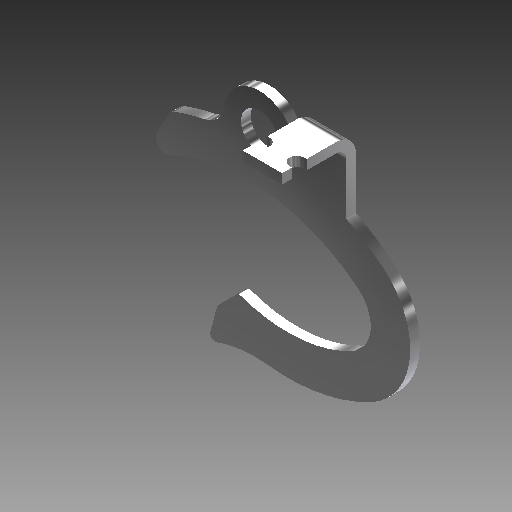
# Autodesk Inventor part: 403-08
Saved by Autodesk Inventor 2019 (Build 230136000, 136)
## iProperties
Company: Autodesk Inc.
Created: 2017-06-27
Part Number: 403-08
Material: Aluminum-6061
Document SubType Name: Sheet Metal
Designer: Autodesk Inc.
Mass: 0.700287 g
Surface Area: 6.63111 cm^2
Volume: 0.259366 cm^3
Density: 2.7 g/cm^3
Sheet Metal Rule: Default_mm
Flat Pattern Width: 2.58001 cm
Flat Pattern Length: 3.04619 cm
Flat Pattern Area: 7.85923 cm^2
Sheet Metal Width: 25.800 mm
Sheet Metal Length: 30.462 mm
Sheet Metal Area: 785.923 mm^2
Appearance: Aluminum - Flat
Author: Inventor
Autodesk Inventor part; units mm, degrees
ref_plane "YZ Plane" through (0, 0, 0) normal (1, 0, 0) x (0, 1, 0)
ref_plane "XZ Plane" through (0, 0, 0) normal (0, 1, 0) x (-1, 0, 0)
ref_plane "XY Plane" through (0, 0, 0) normal (0, 0, 1) x (1, 0, 0)
sketch "Sketch1 outline for Plate1" plane through (0, 0, 0) normal (0, 0, 1) x (1, 0, 0)
  arc A0 (-4.982963, -20.07059) -> (-4.329627, -20.670078) centre (-4.5, -20.2) ccw
  arc A1 (-4.329627, -20.670078) -> (0.795926, -20.076601) centre (-0.513276, -31.19982) cw
  arc A2 (0.795926, -20.076601) -> (11.300243, -18.119671) centre (2.9, -2.2) ccw
  arc A3 (11.300243, -18.119671) -> (12.481249, -5.626677) centre (7.800142, -11.486475) ccw
  arc A4 (12.481249, -5.626677) -> (8.8, -3.245095) centre (-1.25, -22.815417) ccw
  line L0 (8.8, -3.245095) -> (8.8, 3)
  line L1 (8.8, 3) -> (4.8, 3)
  line L2 (4.8, 3) -> (4.8, 1.83303)
  arc A5 (4.8, 1.83303) -> (3.272727, 1.499752) centre (4, 1.83303) cw
  arc A6 (3.272727, 1.499752) -> (-3.571778, 0.449892) centre (0, 0) ccw
  arc A7 (-3.571778, 0.449892) -> (-5.553237, -1.687388) centre (-6.052179, 0.762317) cw
  arc A8 (-5.553237, -1.687388) -> (-8.642869, -2.560617) centre (-1.25, -22.815417) ccw
  arc A9 (-8.642869, -2.560617) -> (-9.177896, -3.021148) centre (-8.3, -3.5) ccw
  line L3 (-9.177896, -3.021148) -> (-10.377896, -5.221148)
  arc A10 (-10.377896, -5.221148) -> (-9.065789, -6.600811) centre (-9.5, -5.7) ccw
  arc A11 (-9.065789, -6.600811) -> (9.984659, -8.751902) centre (-1.25, -22.815417) cw
  arc A12 (9.984659, -8.751902) -> (9.433522, -14.581966) centre (7.800142, -11.486475) cw
  arc A13 (9.433522, -14.581966) -> (-2.131853, -15.264473) centre (2.9, -2.2) cw
  line L4 (-2.131853, -15.264473) -> (-4.26738, -17.4)
  line L5 (-4.26738, -17.4) -> (-4.982963, -20.07059)
extrude "Plate1" add sketch "Sketch1 outline for Plate1" along normal blind 1
sketch "Sketch2 outline for Plate2" plane through (4.8, 3, 0) normal (0, 1, 0) x (1, 0, 0)
  line L0 (4, -5) -> (4, 0)
  line L1 (3.75, -5) -> (4, -5)
  arc A0 (3.75, -6.5) -> (3.75, -5) centre (3.75, -5.75) cw
  line L2 (4, -6.5) -> (3.75, -6.5)
  line L3 (4, -7.5) -> (4, -6.5)
  line L4 (0, -7.5) -> (4, -7.5)
  line L5 (0, -6.5) -> (0, -7.5)
  line L6 (0.25, -6.5) -> (0, -6.5)
  arc A1 (0.25, -5) -> (0.25, -6.5) centre (0.25, -5.75) cw
  line L7 (0, -5) -> (0.25, -5)
  line L8 (0, 0) -> (0, -5)
  line L9 (4, 0) -> (0, 0)
sheet face with bend "Face2" sketch "Sketch2 outline for Plate2" thickness 1 toward (0, 1, 0) bend radius 1
bend "Bend1"
sketch "Sketch1" plane through (0, 0, 0) normal (0, 0, 1) x (1, 0, 0)
  arc A0 (3.272727, 1.499752) -> (-3.571778, 0.449892) centre (0, 0) ccw
  circle A1 centre (-8.3, -3.5) radius 1
  circle A2 centre (-9.5, -5.7) radius 1
  circle A3 centre (-4.5, -20.2) radius 0.5
  arc A4 (9.984659, -8.751902) -> (-9.065789, -6.600811) centre (-1.25, -22.815417) ccw
  line L0 (0, 0) -> (0, -25.191235) construction
  line L1 (-4.982963, -20.07059) -> (-4.26738, -17.4)
  line L2 (-4.26738, -17.4) -> (-2.131853, -15.264473)
  line L3 (-4.26738, -17.4) -> (1.767607, -17.4) construction
  arc A5 (-2.131853, -15.264473) -> (9.433522, -14.581966) centre (2.9, -2.2) ccw
  arc A6 (9.433522, -14.581966) -> (9.984659, -8.751902) centre (7.800142, -11.486475) ccw
  arc A7 (-5.553237, -1.687388) -> (-8.642869, -2.560617) centre (-1.25, -22.815417) ccw
  arc A8 (0.795926, -20.076601) -> (11.300243, -18.119671) centre (2.9, -2.2) ccw
  arc A9 (11.300243, -18.119671) -> (12.481249, -5.626677) centre (7.800142, -11.486475) ccw
  arc A10 (12.481249, -5.626677) -> (8.8, -3.245095) centre (-1.25, -22.815417) ccw
  line L4 (-10.377896, -5.221148) -> (-9.177896, -3.021148)
  arc A11 (0.795926, -20.076601) -> (-4.329627, -20.670078) centre (-0.513276, -31.19982) ccw
  arc A12 (-5.553237, -1.687388) -> (-3.571778, 0.449892) centre (-6.052179, 0.762317) ccw
  line L5 (4.8, 3) -> (8.8, 3)
  line L6 (8.8, 3) -> (8.8, -3.245095)
  arc A13 (3.272727, 1.499752) -> (4.8, 1.83303) centre (4, 1.83303) ccw
  line L7 (4.8, 3) -> (4.8, 1.83303)
  dimension "d34" = 7.2
  dimension "d35" = 2
  dimension "d36" = 8.3
  dimension "d37" = 9.5
  dimension "d38" = 3.5
  dimension "d39" = 5.7
  dimension "d40" = 1
  dimension "d41" = 20.2
  dimension "d42" = 4.5
  dimension "d43" = 1.25
  dimension "d44" = 22.81542
  dimension "d45" = 18
  dimension "d46" = 15
  dimension "d47" = 17.4
  dimension "d48" = 45
  dimension "d49" = 2.9
  dimension "d50" = 2.2
  dimension "d51" = 14
  dimension "d52" = 3.5
  dimension "d53" = 4
  dimension "d54" = 11.2
  dimension "d55" = 2.5
  dimension "d56" = 8.8
  dimension "d57" = 4
  dimension "d58" = 3
  dimension "d59" = 1.6
  dimension "d60" = 18
  dimension "d61" = 22
  measures "d34" diameter of A0
  measures "d35" diameter of A1
  measures "d36" horizontal distance of point (0, 0) A1.centre
  measures "d37" horizontal distance of point (0, 0) A2.centre
  measures "d38" vertical distance of A1.centre point (0, 0)
  measures "d39" vertical distance of L0.start A2.centre
  measures "d40" diameter of A3
  measures "d41" vertical distance of point (0, 0) A3.centre
  measures "d42" horizontal distance of point (0, 0) A3.centre
  measures "d43" horizontal distance of point (0, 0) point (-1.25, -22.815)
  measures "d44" vertical distance of L0.start point (-1.25, -22.815)
  measures "d45" radius of A4
  measures "d46" angle of L0 L1
  measures "d47" vertical distance of point (0, 0) L1.end
  measures "d48" angle of L3 L2
  measures "d49" horizontal distance of point (0, 0) point (2.9, -2.2)
  measures "d50" vertical distance of point (0, 0) point (2.9, -2.2)
  measures "d51" radius of A5
  measures "d52" radius of A6
  measures "d53" radial gap between concentric circles of A9 A6
  measures "d54" radius of A11
  measures "d55" radius of A12
  measures "d56" horizontal distance of L0.start L5.end
  measures "d57" distance of L5.start L5.end
  measures "d58" distance from line of L5 L0.start
  measures "d59" diameter of A13
  measures "d60" radius of A8
  measures "d61" radius of A10
sketch "Sketch2" plane through (4.8, 3, 0) normal (0, 1, 0) x (1, 0, 0)
  line L0 (4, 0) -> (0, 0)
  line L1 (4, 0) -> (0, 0)
  line L2 (0, 0) -> (0, -7.5)
  line L3 (0, -7.5) -> (4, -7.5)
  line L4 (4, -7.5) -> (4, 0)
  line L5 (0, -6.5) -> (0.25, -6.5)
  arc A0 (0.25, -6.5) -> (0.25, -5) centre (0.25, -5.75) ccw
  line L6 (0.25, -5) -> (0, -5)
  line L7 (4, -6.5) -> (3.75, -6.5)
  arc A1 (3.75, -5) -> (3.75, -6.5) centre (3.75, -5.75) ccw
  line L8 (3.75, -5) -> (4, -5)
  line L9 (0, -1) -> (4, -1)
  point P0 (-4.8, 0)
  dimension "d65" = 0.75
  dimension "d66" = 3.5
  dimension "d84" = 6.5
  dimension "d85" = 4.75
  measures "d65" radius of A0
  measures "d66" distance of A1.centre A0.centre
  measures "d84" distance between parallel lines of L3 L9
  measures "d85" distance from line of A1.centre L9
hole "Hole1" at (0, 0, 1) direction (0, 0, -1) diameter 3.75 end through all
fillet "Fillet1" radius 0.5 2 edges at (-4.2674, -17.4, 0.5) (-2.1319, -15.2645, 0.5)
equation "\"d81\" = Thickness"
equation "\"d86\" = Thickness"
equation "\"d69\" = BendRadius"
equation "\"d70\" = BendReliefWidth"
equation "\"d72\" = MinimumRemnant"
equation "\"d71\" = BendReliefDepth"
equation "\"d73\" = BendRadius"
equation "\"BendRadius\" = Thickness"
equation "\"BendReliefWidth\" = Thickness"
equation "\"BendReliefDepth\" = 0.5 * Thickness"
equation "\"CornerReliefSize\" = 4 * Thickness"
equation "\"MinimumRemnant\" = 2 * Thickness"
equation "\"TransitionRadius\" = BendRadius"
equation "\"JacobiRadiusSize\" = BendRadius"
equation "\"GapSize\" = Thickness"
equation "\"d62\" = BendRadius"
equation "\"Thickness\" = 1"
body "Solid1"
